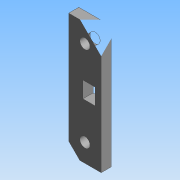
# Autodesk Inventor part: holder_sideblock
Saved by Autodesk Inventor 2015 (Build 190159000, 159)
## iProperties
Created: 2014-09-02
Part Number: holder_sideblock
Material: Generic
Document SubType Name: Modeling
Designer: shohei
Density: 1 g/cm^3
Appearance: Default
Author: shohei
Autodesk Inventor part; units mm, degrees
ref_plane "YZ Plane" through (0, 0, 0) normal (1, 0, 0) x (0, 1, 0)
ref_plane "XZ Plane" through (0, 0, 0) normal (0, 1, 0) x (-1, 0, 0)
ref_plane "XY Plane" through (0, 0, 0) normal (0, 0, 1) x (1, 0, 0)
sketch "Sketch1" plane through (0, 0, 0) normal (0, 1, 0) x (-1, 0, 0)
  line L0 (0, 0) -> (16, 0)
  line L1 (16, 0) -> (16, 60)
  line L2 (16, 60) -> (0, 60)
  line L3 (0, 60) -> (0, 0)
  circle A0 centre (8, 51) radius 2.5
  circle A1 centre (8, 9) radius 2.5
  dimension "d2" = 60
  dimension "d3" = 16
  dimension "d4" = 8
  dimension "d5" = 5
  dimension "d6" = 9
  dimension "d7" = 8
  dimension "d8" = 9
  dimension "d9" = 5
  constraints: 8 end point, 2 centre point, 2 parallel, 1 horizontal, 1 perpendicular
  measures "d2" distance of L0.end L1.end
  measures "d3" distance of L1.end L2.end
  measures "d4" distance from line of L1 A0.centre
  measures "d5" diameter of A0
  measures "d6" distance from line of L2 A0.centre
  measures "d7" distance from line of L1 A1.centre
  measures "d8" distance from line of L0 A1.centre
  measures "d9" diameter of A1
extrude "Extrusion1" add sketch "Sketch1" along normal blind 5
sketch "Sketch2" plane through (0, 5, 0) normal (0, 1, 0) x (1, 0, 0)
  line L0 (-9, -27) -> (-3, -27)
  line L1 (-3, -27) -> (-3, -35)
  line L2 (-3, -35) -> (-9, -35)
  line L3 (-9, -35) -> (-9, -27)
  line L4 (-16, 0) -> (-16, -60) projected
  line L5 (-16, -60) -> (0, -60) projected
  point P0 (0, 0)
  dimension "d10" = 8
  dimension "d11" = 6
  dimension "d12" = 7
  dimension "d13" = 25
  constraints: 8 end point, 2 parallel, 1 horizontal, 1 perpendicular
  measures "d10" distance of L2.end L0.start
  measures "d11" distance of L0.start L0.end
  measures "d12" distance between parallel lines of L4 L3
  measures "d13" distance between parallel lines of L5 L2
extrude "Extrusion2" cut sketch "Sketch2" against normal through all
body "Solid1"
